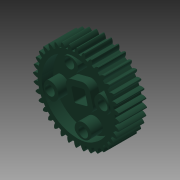
# Autodesk Inventor part: High Strength 36 Tooth Gear
Saved by Autodesk Inventor 2016 SP2 (Build 200236200, 236)
## iProperties
Category: Motion
Company: Autodesk Inc.
Created: 2012-02-19
Part Number: High Strength 36 Tooth Gear
Document SubType Name: Modeling
Designer: Autodesk Inc.
Density: 1.42 g/cm^3
Catalog Web Link: http://www.vexrobotics.com/276-2250.html
Description: 36 tooth spur gear
Vendor: VEX
Material: Acetal Resin, White
Mass: 10.4214 g
Surface Area: 82.0542 cm^2
Volume: 7.33901 cm^3
Appearance: VEX Gears Green
Author: Autodesk Inc.
Autodesk Inventor part; units mm, degrees
sketch "Sketch1" plane through (0, 0, 0) normal (0, 0, 1) x (1, 0, 0)
  arc A0 (-19.7463, 3.7758) -> (-19.8092, 3.4306) centre (0, 0) ccw
  arc A1 (-19.8092, 3.4306) -> (-17.8392, 2.2932) centre (-17.463, 5.2196) ccw
  arc A2 (-17.8392, 2.2932) -> (-17.9557, 1.0433) centre (0, 0) ccw
  arc A3 (-17.9557, 1.0433) -> (-20.102, 0.2896) centre (-18.1269, -1.9022) ccw
  arc A4 (-20.102, 0.2896) -> (-20.104, -0.0613) centre (0, 0) ccw
  arc A5 (-20.104, -0.0613) -> (-17.9664, -0.8393) centre (-18.1041, 2.1079) ccw
  arc A6 (-17.9664, -0.8393) -> (-17.8641, -2.0906) centre (0, 0) ccw
  arc A7 (-17.8641, -2.0906) -> (-19.8469, -3.2055) centre (-17.5212, -5.021) ccw
  arc A8 (-19.8469, -3.2055) -> (-19.7879, -3.5514) centre (0, 0) ccw
  arc A9 (-19.7879, -3.5514) -> (-17.5477, -3.9464) centre (-18.1951, -1.0679) ccw
  arc A10 (-17.5477, -3.9464) -> (-17.2297, -5.1609) centre (0, 0) ccw
  arc A11 (-17.2297, -5.1609) -> (-18.9887, -6.6032) centre (-16.3831, -7.9872) ccw
  arc A12 (-18.9887, -6.6032) -> (-18.8706, -6.9336) centre (0, 0) ccw
  arc A13 (-18.8706, -6.9336) -> (-16.5958, -6.9336) centre (-17.7332, -4.2112) ccw
  arc A14 (-16.5958, -6.9336) -> (-16.0717, -8.0744) centre (0, 0) ccw
  arc A15 (-16.0717, -8.0744) -> (-17.5536, -9.8002) centre (-14.7472, -10.7108) ccw
  arc A16 (-17.5536, -9.8002) -> (-17.3799, -10.1051) centre (0, 0) ccw
  arc A17 (-17.3799, -10.1051) -> (-15.1397, -9.7101) centre (-16.7325, -7.2266) ccw
  arc A18 (-15.1397, -9.7101) -> (-14.4255, -10.7425) centre (0, 0) ccw
  arc A19 (-14.4255, -10.7425) -> (-15.5852, -12.6995) centre (-12.6633, -13.1089) ccw
  arc A20 (-15.5852, -12.6995) -> (-15.3612, -12.9696) centre (0, 0) ccw
  arc A21 (-15.3612, -12.9696) -> (-13.2236, -12.1916) centre (-15.2235, -10.0223) ccw
  arc A22 (-13.2236, -12.1916) -> (-12.3409, -13.0843) centre (0, 0) ccw
  arc A23 (-12.3409, -13.0843) -> (-13.1431, -15.2129) centre (-10.1945, -15.1087) ccw
  arc A24 (-13.1431, -15.2129) -> (-12.8756, -15.44) centre (0, 0) ccw
  arc A25 (-12.8756, -15.44) -> (-10.9056, -14.3026) centre (-13.2518, -12.5136) ccw
  arc A26 (-10.9056, -14.3026) -> (-9.8814, -15.0285) centre (0, 0) ccw
  arc A27 (-9.8814, -15.0285) -> (-10.3018, -17.2641) centre (-7.4161, -16.6494) ccw
  arc A28 (-10.3018, -17.2641) -> (-9.9989, -17.4412) centre (0, 0) ccw
  arc A29 (-9.9989, -17.4412) -> (-8.2563, -15.979) centre (-10.8775, -14.6247) ccw
  arc A30 (-8.2563, -15.979) -> (-7.1216, -16.516) centre (0, 0) ccw
  arc A31 (-7.1216, -16.516) -> (-7.1474, -18.7907) centre (-4.4123, -17.6843) ccw
  arc A32 (-7.1474, -18.7907) -> (-6.8184, -18.9126) centre (0, 0) ccw
  arc A33 (-6.8184, -18.9126) -> (-5.3562, -17.17) centre (-8.1727, -16.2913) ccw
  arc A34 (-5.3562, -17.17) -> (-4.1454, -17.5018) centre (0, 0) ccw
  arc A35 (-4.1454, -17.5018) -> (-3.7758, -19.7463) centre (-1.2744, -18.1818) ccw
  arc A36 (-3.7758, -19.7463) -> (-3.4306, -19.8092) centre (0, 0) ccw
  arc A37 (-3.4306, -19.8092) -> (-2.2932, -17.8392) centre (-5.2196, -17.463) ccw
  arc A38 (-2.2932, -17.8392) -> (-1.0433, -17.9557) centre (0, 0) ccw
  arc A39 (-1.0433, -17.9557) -> (-0.2896, -20.102) centre (1.9022, -18.1269) ccw
  arc A40 (-0.2896, -20.102) -> (0.0613, -20.104) centre (0, 0) ccw
  arc A41 (0.0613, -20.104) -> (0.8393, -17.9664) centre (-2.1079, -18.1041) ccw
  arc A42 (0.8393, -17.9664) -> (2.0906, -17.8641) centre (0, 0) ccw
  arc A43 (2.0906, -17.8641) -> (3.2055, -19.8469) centre (5.021, -17.5212) ccw
  arc A44 (3.2055, -19.8469) -> (3.5514, -19.7879) centre (0, 0) ccw
  arc A45 (3.5514, -19.7879) -> (3.9464, -17.5477) centre (1.0679, -18.1951) ccw
  arc A46 (3.9464, -17.5477) -> (5.1609, -17.2297) centre (0, 0) ccw
  arc A47 (5.1609, -17.2297) -> (6.6032, -18.9887) centre (7.9872, -16.3831) ccw
  arc A48 (6.6032, -18.9887) -> (6.9336, -18.8706) centre (0, 0) ccw
  arc A49 (6.9336, -18.8706) -> (6.9336, -16.5958) centre (4.2112, -17.7332) ccw
  arc A50 (6.9336, -16.5958) -> (8.0744, -16.0717) centre (0, 0) ccw
  arc A51 (8.0744, -16.0717) -> (9.8002, -17.5536) centre (10.7108, -14.7472) ccw
  arc A52 (9.8002, -17.5536) -> (10.1051, -17.3799) centre (0, 0) ccw
  arc A53 (10.1051, -17.3799) -> (9.7101, -15.1397) centre (7.2266, -16.7325) ccw
  arc A54 (9.7101, -15.1397) -> (10.7425, -14.4255) centre (0, 0) ccw
  arc A55 (10.7425, -14.4255) -> (12.6995, -15.5852) centre (13.1089, -12.6633) ccw
  arc A56 (12.6995, -15.5852) -> (12.9696, -15.3612) centre (0, 0) ccw
  arc A57 (12.9696, -15.3612) -> (12.1916, -13.2236) centre (10.0223, -15.2235) ccw
  arc A58 (12.1916, -13.2236) -> (13.0843, -12.3409) centre (0, 0) ccw
  arc A59 (13.0843, -12.3409) -> (15.2129, -13.1431) centre (15.1087, -10.1945) ccw
  arc A60 (15.2129, -13.1431) -> (15.44, -12.8756) centre (0, 0) ccw
  arc A61 (15.44, -12.8756) -> (14.3026, -10.9056) centre (12.5136, -13.2518) ccw
  arc A62 (14.3026, -10.9056) -> (15.0285, -9.8814) centre (0, 0) ccw
  arc A63 (15.0285, -9.8814) -> (17.2641, -10.3018) centre (16.6494, -7.4161) ccw
  arc A64 (17.2641, -10.3018) -> (17.4412, -9.9989) centre (0, 0) ccw
  arc A65 (17.4412, -9.9989) -> (15.979, -8.2563) centre (14.6247, -10.8775) ccw
  arc A66 (15.979, -8.2563) -> (16.516, -7.1216) centre (0, 0) ccw
  arc A67 (16.516, -7.1216) -> (18.7907, -7.1474) centre (17.6843, -4.4123) ccw
  arc A68 (18.7907, -7.1474) -> (18.9126, -6.8184) centre (0, 0) ccw
  arc A69 (18.9126, -6.8184) -> (17.17, -5.3562) centre (16.2913, -8.1727) ccw
  arc A70 (17.17, -5.3562) -> (17.5018, -4.1454) centre (0, 0) ccw
  arc A71 (17.5018, -4.1454) -> (19.7463, -3.7758) centre (18.1818, -1.2744) ccw
  arc A72 (19.7463, -3.7758) -> (19.8092, -3.4306) centre (0, 0) ccw
  arc A73 (19.8092, -3.4306) -> (17.8392, -2.2932) centre (17.463, -5.2196) ccw
  arc A74 (17.8392, -2.2932) -> (17.9557, -1.0433) centre (0, 0) ccw
  arc A75 (17.9557, -1.0433) -> (20.102, -0.2896) centre (18.1269, 1.9022) ccw
  arc A76 (20.102, -0.2896) -> (20.104, 0.0613) centre (0, 0) ccw
  arc A77 (20.104, 0.0613) -> (17.9664, 0.8393) centre (18.1041, -2.1079) ccw
  arc A78 (17.9664, 0.8393) -> (17.8641, 2.0906) centre (0, 0) ccw
  arc A79 (17.8641, 2.0906) -> (19.8469, 3.2055) centre (17.5212, 5.021) ccw
  arc A80 (19.8469, 3.2055) -> (19.7879, 3.5514) centre (0, 0) ccw
  arc A81 (19.7879, 3.5514) -> (17.5477, 3.9464) centre (18.1951, 1.0679) ccw
  arc A82 (17.5477, 3.9464) -> (17.2297, 5.1609) centre (0, 0) ccw
  arc A83 (17.2297, 5.1609) -> (18.9887, 6.6032) centre (16.3831, 7.9872) ccw
  arc A84 (18.9887, 6.6032) -> (18.8706, 6.9336) centre (0, 0) ccw
  arc A85 (18.8706, 6.9336) -> (16.5958, 6.9336) centre (17.7332, 4.2112) ccw
  arc A86 (16.5958, 6.9336) -> (16.0717, 8.0744) centre (0, 0) ccw
  arc A87 (16.0717, 8.0744) -> (17.5536, 9.8002) centre (14.7472, 10.7108) ccw
  arc A88 (17.5536, 9.8002) -> (17.3799, 10.1051) centre (0, 0) ccw
  arc A89 (17.3799, 10.1051) -> (15.1397, 9.7101) centre (16.7325, 7.2266) ccw
  arc A90 (15.1397, 9.7101) -> (14.4255, 10.7425) centre (0, 0) ccw
  arc A91 (14.4255, 10.7425) -> (15.5852, 12.6995) centre (12.6633, 13.1089) ccw
  arc A92 (15.5852, 12.6995) -> (15.3612, 12.9696) centre (0, 0) ccw
  arc A93 (15.3612, 12.9696) -> (13.2235, 12.1916) centre (15.2235, 10.0223) ccw
  arc A94 (13.2235, 12.1916) -> (12.3409, 13.0843) centre (0, 0) ccw
  arc A95 (12.3409, 13.0843) -> (13.1431, 15.2129) centre (10.1945, 15.1087) ccw
  arc A96 (13.1431, 15.2129) -> (12.8756, 15.44) centre (0, 0) ccw
  arc A97 (12.8756, 15.44) -> (10.9056, 14.3026) centre (13.2518, 12.5136) ccw
  arc A98 (10.9056, 14.3026) -> (9.8814, 15.0285) centre (0, 0) ccw
  arc A99 (9.8814, 15.0285) -> (10.3018, 17.2641) centre (7.4161, 16.6494) ccw
  arc A100 (10.3018, 17.2641) -> (9.9989, 17.4412) centre (0, 0) ccw
  arc A101 (9.9989, 17.4412) -> (8.2563, 15.979) centre (10.8775, 14.6247) ccw
  arc A102 (8.2563, 15.979) -> (7.1216, 16.516) centre (0, 0) ccw
  arc A103 (7.1216, 16.516) -> (7.1474, 18.7907) centre (4.4123, 17.6843) ccw
  arc A104 (7.1474, 18.7907) -> (6.8184, 18.9126) centre (0, 0) ccw
  arc A105 (6.8184, 18.9126) -> (5.3562, 17.17) centre (8.1727, 16.2913) ccw
  arc A106 (5.3562, 17.17) -> (4.1454, 17.5018) centre (0, 0) ccw
  arc A107 (4.1454, 17.5018) -> (3.7758, 19.7463) centre (1.2744, 18.1818) ccw
  arc A108 (3.7758, 19.7463) -> (3.4306, 19.8092) centre (0, 0) ccw
  arc A109 (3.4306, 19.8092) -> (2.2932, 17.8392) centre (5.2196, 17.463) ccw
  arc A110 (2.2932, 17.8392) -> (1.0433, 17.9557) centre (0, 0) ccw
  arc A111 (1.0433, 17.9557) -> (0.2896, 20.102) centre (-1.9022, 18.1269) ccw
  arc A112 (0.2896, 20.102) -> (-0.0613, 20.104) centre (0, 0) ccw
  arc A113 (-0.0613, 20.104) -> (-0.8393, 17.9664) centre (2.1079, 18.1041) ccw
  arc A114 (-0.8393, 17.9664) -> (-2.0906, 17.8641) centre (0, 0) ccw
  arc A115 (-2.0906, 17.8641) -> (-3.2055, 19.8469) centre (-5.021, 17.5212) ccw
  arc A116 (-3.2055, 19.8469) -> (-3.5514, 19.7879) centre (0, 0) ccw
  arc A117 (-3.5514, 19.7879) -> (-3.9464, 17.5477) centre (-1.0679, 18.1951) ccw
  arc A118 (-3.9464, 17.5477) -> (-5.1609, 17.2297) centre (0, 0) ccw
  arc A119 (-5.1609, 17.2297) -> (-6.6032, 18.9888) centre (-7.9872, 16.3831) ccw
  arc A120 (-6.6032, 18.9888) -> (-6.9336, 18.8706) centre (0, 0) ccw
  arc A121 (-6.9336, 18.8706) -> (-6.9336, 16.5958) centre (-4.2112, 17.7332) ccw
  arc A122 (-6.9336, 16.5958) -> (-8.0744, 16.0717) centre (0, 0) ccw
  arc A123 (-8.0744, 16.0717) -> (-9.8002, 17.5536) centre (-10.7108, 14.7472) ccw
  arc A124 (-9.8002, 17.5536) -> (-10.1051, 17.3799) centre (0, 0) ccw
  arc A125 (-10.1051, 17.3799) -> (-9.7101, 15.1397) centre (-7.2266, 16.7325) ccw
  arc A126 (-9.7101, 15.1397) -> (-10.7425, 14.4255) centre (0, 0) ccw
  arc A127 (-10.7425, 14.4255) -> (-12.6995, 15.5852) centre (-13.1089, 12.6633) ccw
  arc A128 (-12.6995, 15.5852) -> (-12.9696, 15.3612) centre (0, 0) ccw
  arc A129 (-12.9696, 15.3612) -> (-12.1916, 13.2236) centre (-10.0223, 15.2235) ccw
  arc A130 (-12.1916, 13.2236) -> (-13.0843, 12.3409) centre (0, 0) ccw
  arc A131 (-13.0843, 12.3409) -> (-15.2129, 13.1431) centre (-15.1087, 10.1945) ccw
  arc A132 (-15.2129, 13.1431) -> (-15.44, 12.8756) centre (0, 0) ccw
  arc A133 (-15.44, 12.8756) -> (-14.3026, 10.9056) centre (-12.5136, 13.2518) ccw
  arc A134 (-14.3026, 10.9056) -> (-15.0285, 9.8814) centre (0, 0) ccw
  arc A135 (-15.0285, 9.8814) -> (-17.2641, 10.3018) centre (-16.6494, 7.4161) ccw
  arc A136 (-17.2641, 10.3018) -> (-17.4412, 9.9989) centre (0, 0) ccw
  arc A137 (-17.4412, 9.9989) -> (-15.979, 8.2563) centre (-14.6247, 10.8775) ccw
  arc A138 (-15.979, 8.2563) -> (-16.516, 7.1216) centre (0, 0) ccw
  arc A139 (-16.516, 7.1216) -> (-18.7907, 7.1474) centre (-17.6843, 4.4123) ccw
  arc A140 (-18.7907, 7.1474) -> (-18.9126, 6.8184) centre (0, 0) ccw
  arc A141 (-18.9126, 6.8184) -> (-17.17, 5.3562) centre (-16.2913, 8.1727) ccw
  arc A142 (-17.17, 5.3562) -> (-17.5018, 4.1454) centre (0, 0) ccw
  arc A143 (-17.5018, 4.1454) -> (-19.7463, 3.7758) centre (-18.1818, 1.2744) ccw
  arc A144 (-8.6835, 13.422) -> (-15.9553, 0.9903) centre (0, 0) ccw
  arc A145 (0.9903, 15.9553) -> (-8.6835, 13.422) centre (-0.8133, 3.1059) ccw
  arc A146 (13.422, 8.6835) -> (0.9903, 15.9553) centre (0, 0) ccw
  arc A147 (15.9553, -0.9903) -> (13.422, 8.6835) centre (3.1059, 0.8133) ccw
  arc A148 (8.6835, -13.422) -> (15.9553, -0.9903) centre (0, 0) ccw
  arc A149 (-0.9903, -15.9553) -> (8.6835, -13.422) centre (0.8133, -3.1059) ccw
  arc A150 (-13.422, -8.6835) -> (-0.9903, -15.9553) centre (0, 0) ccw
  arc A151 (-15.9553, 0.9903) -> (-13.422, -8.6835) centre (-3.1059, -0.8133) ccw
  line L0 (0.9929, 6.2349) -> (-3.9214, 4.948)
  arc A152 (-3.9214, 4.948) -> (-6.2349, 0.9929) centre (-3.1006, 1.8137) ccw
  line L1 (-6.2349, 0.9929) -> (-4.948, -3.9214)
  arc A153 (-4.948, -3.9214) -> (-0.9929, -6.2349) centre (-1.8137, -3.1006) ccw
  line L2 (-0.9929, -6.2349) -> (3.9214, -4.948)
  arc A154 (3.9214, -4.948) -> (6.2349, -0.9929) centre (3.1006, -1.8137) ccw
  line L3 (6.2349, -0.9929) -> (4.948, 3.9214)
  arc A155 (4.948, 3.9214) -> (0.9929, 6.2349) centre (1.8137, 3.1006) ccw
  arc A156 (-3.2615, 2.428) -> (-3.7149, 1.6528) centre (-3.1006, 1.8137) ccw
  line L4 (-3.2615, 2.428) -> (1.6528, 3.7149)
  arc A157 (2.428, 3.2615) -> (1.6528, 3.7149) centre (1.8137, 3.1006) ccw
  line L5 (2.428, 3.2615) -> (3.7149, -1.6528)
  arc A158 (3.2615, -2.428) -> (3.7149, -1.6528) centre (3.1006, -1.8137) ccw
  line L6 (3.2615, -2.428) -> (-1.6528, -3.7149)
  arc A159 (-2.428, -3.2615) -> (-1.6528, -3.7149) centre (-1.8137, -3.1006) ccw
  line L7 (-2.428, -3.2615) -> (-3.7149, 1.6528)
  arc A160 (-0.6522, -13.299) -> (7.0868, -11.2724) centre (2.8806, -11.0001) ccw
  arc A161 (7.0868, -11.2724) -> (-0.6522, -13.299) centre (3.2173, -12.2857) ccw
  circle A162 centre (3.2173, -12.2857) radius 2.2225
  arc A163 (-13.299, 0.6522) -> (-11.2724, -7.0868) centre (-11.0001, -2.8806) ccw
  arc A164 (-11.2724, -7.0868) -> (-13.299, 0.6522) centre (-12.2857, -3.2173) ccw
  circle A165 centre (-12.2857, -3.2173) radius 2.2225
  arc A166 (0.6522, 13.299) -> (-7.0868, 11.2724) centre (-2.8806, 11.0001) ccw
  arc A167 (-7.0868, 11.2724) -> (0.6522, 13.299) centre (-3.2173, 12.2857) ccw
  circle A168 centre (-3.2173, 12.2857) radius 2.2225
  arc A169 (13.299, -0.6522) -> (11.2724, 7.0868) centre (11.0001, 2.8806) ccw
  arc A170 (11.2724, 7.0868) -> (13.299, -0.6522) centre (12.2857, 3.2173) ccw
  circle A171 centre (12.2857, 3.2173) radius 2.2225
  point P0 (0, 0)
  constraints: 336 point on circle, 172 centre point, 16 end point
extrude "Extrusion1" add sketch "Sketch1" against normal blind 12.7 contours A143 A142 A141 A140 A139 A138 A137 A136 A135 A134 A133 A132 A131 A130 A129 A128 A127 A126 A125 A124 A123 A122 A121 A120 A119 A118 A117 A116 A115 A114 A113 A112 A111 A110 A109 A108 A107 A106 A105 A104 A103 A102 A101 A100 A99 A98 A97 A96 A95 A94 A93 A92 A91 A90 A89 A88 A87 A86 A85 A84 A83 A82 A81 A80 A79 A78 A77 A76 A75 A74 A73 A72 A71 A70 A69 A68 A67 A66 A65 A64 A63 A62 A61 A60 A59 A58 A57 A56 A55 A54 A53 A52 A51 A50 A49 A48 A47 A46 A45 A44 A43 A42 A41 A40 A39 A38 A37 A36 A35 A34 A33 A32 A31 A30 A29 A28 A27 A26 A25 A24 A23 A22 A21 A20 A19 A18 A17 A16 A15 A14 A13 A12 A11 A10 A9 A8 A7 A6 A5 A4 A3 A2 A1 A0
ref_plane "Work Plane1" through (0, 0, -6.35) normal (0, 0, 1) x (1, 0, 0)
sketch "Sketch2" plane through (0, 0, -6.35) normal (0, 0, 1) x (1, 0, 0)
  arc A0 (-15.9553, 0.9903) -> (-13.422, -8.6835) centre (-3.1059, -0.8133) ccw projected
  arc A1 (-13.422, -8.6835) -> (-0.9903, -15.9553) centre (0, 0) ccw projected
  arc A2 (-0.9903, -15.9553) -> (8.6835, -13.422) centre (0.8133, -3.1059) ccw projected
  arc A3 (8.6835, -13.422) -> (15.9553, -0.9903) centre (0, 0) ccw projected
  arc A4 (15.9553, -0.9903) -> (13.422, 8.6835) centre (3.1059, 0.8133) ccw projected
  arc A5 (13.422, 8.6835) -> (0.9903, 15.9553) centre (0, 0) ccw projected
  arc A6 (0.9903, 15.9553) -> (-8.6835, 13.422) centre (-0.8133, 3.1059) ccw projected
  arc A7 (-8.6835, 13.422) -> (-15.9553, 0.9903) centre (0, 0) ccw projected
  arc A8 (-15.979, 8.2563) -> (-16.516, 7.1216) centre (0, 0) ccw projected
  arc A9 (-17.4412, 9.9989) -> (-15.979, 8.2563) centre (-14.6247, 10.8775) ccw projected
  arc A10 (-17.2641, 10.3018) -> (-17.4412, 9.9989) centre (0, 0) ccw projected
  arc A11 (-15.0285, 9.8814) -> (-17.2641, 10.3018) centre (-16.6494, 7.4161) ccw projected
  arc A12 (-14.3026, 10.9056) -> (-15.0285, 9.8814) centre (0, 0) ccw projected
  arc A13 (-15.44, 12.8756) -> (-14.3026, 10.9056) centre (-12.5136, 13.2518) ccw projected
  arc A14 (-15.2129, 13.1431) -> (-15.44, 12.8756) centre (0, 0) ccw projected
  arc A15 (-13.0843, 12.3409) -> (-15.2129, 13.1431) centre (-15.1087, 10.1945) ccw projected
  arc A16 (-12.1916, 13.2236) -> (-13.0843, 12.3409) centre (0, 0) ccw projected
  arc A17 (-12.9696, 15.3612) -> (-12.1916, 13.2236) centre (-10.0223, 15.2235) ccw projected
  arc A18 (-12.6995, 15.5852) -> (-12.9696, 15.3612) centre (0, 0) ccw projected
  arc A19 (-10.7425, 14.4255) -> (-12.6995, 15.5852) centre (-13.1089, 12.6633) ccw projected
  arc A20 (-9.7101, 15.1397) -> (-10.7425, 14.4255) centre (0, 0) ccw projected
  arc A21 (-10.1051, 17.3799) -> (-9.7101, 15.1397) centre (-7.2266, 16.7325) ccw projected
  arc A22 (-9.8002, 17.5536) -> (-10.1051, 17.3799) centre (0, 0) ccw projected
  arc A23 (-8.0744, 16.0717) -> (-9.8002, 17.5536) centre (-10.7108, 14.7472) ccw projected
  arc A24 (-6.9336, 16.5958) -> (-8.0744, 16.0717) centre (0, 0) ccw projected
  arc A25 (-6.9336, 18.8706) -> (-6.9336, 16.5958) centre (-4.2112, 17.7332) ccw projected
  arc A26 (-6.6032, 18.9888) -> (-6.9336, 18.8706) centre (0, 0) ccw projected
  arc A27 (-5.1609, 17.2297) -> (-6.6032, 18.9888) centre (-7.9872, 16.3831) ccw projected
  arc A28 (-3.9464, 17.5477) -> (-5.1609, 17.2297) centre (0, 0) ccw projected
  arc A29 (-3.5514, 19.7879) -> (-3.9464, 17.5477) centre (-1.0679, 18.1951) ccw projected
  arc A30 (-3.2055, 19.8469) -> (-3.5514, 19.7879) centre (0, 0) ccw projected
  arc A31 (-2.0906, 17.8641) -> (-3.2055, 19.8469) centre (-5.021, 17.5212) ccw projected
  arc A32 (-0.8393, 17.9664) -> (-2.0906, 17.8641) centre (0, 0) ccw projected
  arc A33 (-0.0613, 20.104) -> (-0.8393, 17.9664) centre (2.1079, 18.1041) ccw projected
  arc A34 (0.2896, 20.102) -> (-0.0613, 20.104) centre (0, 0) ccw projected
  arc A35 (1.0433, 17.9557) -> (0.2896, 20.102) centre (-1.9022, 18.1269) ccw projected
  arc A36 (2.2932, 17.8392) -> (1.0433, 17.9557) centre (0, 0) ccw projected
  arc A37 (3.4306, 19.8092) -> (2.2932, 17.8392) centre (5.2196, 17.463) ccw projected
  arc A38 (3.7758, 19.7463) -> (3.4306, 19.8092) centre (0, 0) ccw projected
  arc A39 (4.1454, 17.5018) -> (3.7758, 19.7463) centre (1.2744, 18.1818) ccw projected
  arc A40 (5.3562, 17.17) -> (4.1454, 17.5018) centre (0, 0) ccw projected
  arc A41 (6.8184, 18.9126) -> (5.3562, 17.17) centre (8.1727, 16.2913) ccw projected
  arc A42 (7.1474, 18.7907) -> (6.8184, 18.9126) centre (0, 0) ccw projected
  arc A43 (7.1216, 16.516) -> (7.1474, 18.7907) centre (4.4123, 17.6843) ccw projected
  arc A44 (8.2563, 15.979) -> (7.1216, 16.516) centre (0, 0) ccw projected
  arc A45 (9.9989, 17.4412) -> (8.2563, 15.979) centre (10.8775, 14.6247) ccw projected
  arc A46 (10.3018, 17.2641) -> (9.9989, 17.4412) centre (0, 0) ccw projected
  arc A47 (9.8814, 15.0285) -> (10.3018, 17.2641) centre (7.4161, 16.6494) ccw projected
  arc A48 (10.9056, 14.3026) -> (9.8814, 15.0285) centre (0, 0) ccw projected
  arc A49 (12.8756, 15.44) -> (10.9056, 14.3026) centre (13.2518, 12.5136) ccw projected
  arc A50 (13.1431, 15.2129) -> (12.8756, 15.44) centre (0, 0) ccw projected
  arc A51 (12.3409, 13.0843) -> (13.1431, 15.2129) centre (10.1945, 15.1087) ccw projected
  arc A52 (13.2235, 12.1916) -> (12.3409, 13.0843) centre (0, 0) ccw projected
  arc A53 (15.3612, 12.9696) -> (13.2235, 12.1916) centre (15.2235, 10.0223) ccw projected
  arc A54 (15.5852, 12.6995) -> (15.3612, 12.9696) centre (0, 0) ccw projected
  arc A55 (14.4255, 10.7425) -> (15.5852, 12.6995) centre (12.6633, 13.1089) ccw projected
  arc A56 (15.1397, 9.7101) -> (14.4255, 10.7425) centre (0, 0) ccw projected
  arc A57 (17.3799, 10.1051) -> (15.1397, 9.7101) centre (16.7325, 7.2266) ccw projected
  arc A58 (17.5536, 9.8002) -> (17.3799, 10.1051) centre (0, 0) ccw projected
  arc A59 (16.0717, 8.0744) -> (17.5536, 9.8002) centre (14.7472, 10.7108) ccw projected
  arc A60 (16.5958, 6.9336) -> (16.0717, 8.0744) centre (0, 0) ccw projected
  arc A61 (18.8706, 6.9336) -> (16.5958, 6.9336) centre (17.7332, 4.2112) ccw projected
  arc A62 (18.9887, 6.6032) -> (18.8706, 6.9336) centre (0, 0) ccw projected
  arc A63 (17.2297, 5.1609) -> (18.9887, 6.6032) centre (16.3831, 7.9872) ccw projected
  arc A64 (17.5477, 3.9464) -> (17.2297, 5.1609) centre (0, 0) ccw projected
  arc A65 (19.7879, 3.5514) -> (17.5477, 3.9464) centre (18.1951, 1.0679) ccw projected
  arc A66 (19.8469, 3.2055) -> (19.7879, 3.5514) centre (0, 0) ccw projected
  arc A67 (17.8641, 2.0906) -> (19.8469, 3.2055) centre (17.5212, 5.021) ccw projected
  arc A68 (17.9664, 0.8393) -> (17.8641, 2.0906) centre (0, 0) ccw projected
  arc A69 (20.104, 0.0613) -> (17.9664, 0.8393) centre (18.1041, -2.1079) ccw projected
  arc A70 (20.102, -0.2896) -> (20.104, 0.0613) centre (0, 0) ccw projected
  arc A71 (17.9557, -1.0433) -> (20.102, -0.2896) centre (18.1269, 1.9022) ccw projected
  arc A72 (17.8392, -2.2932) -> (17.9557, -1.0433) centre (0, 0) ccw projected
  arc A73 (19.8092, -3.4306) -> (17.8392, -2.2932) centre (17.463, -5.2196) ccw projected
  arc A74 (19.7463, -3.7758) -> (19.8092, -3.4306) centre (0, 0) ccw projected
  arc A75 (17.5018, -4.1454) -> (19.7463, -3.7758) centre (18.1818, -1.2744) ccw projected
  arc A76 (17.17, -5.3562) -> (17.5018, -4.1454) centre (0, 0) ccw projected
  arc A77 (18.9126, -6.8184) -> (17.17, -5.3562) centre (16.2913, -8.1727) ccw projected
  arc A78 (18.7907, -7.1474) -> (18.9126, -6.8184) centre (0, 0) ccw projected
  arc A79 (16.516, -7.1216) -> (18.7907, -7.1474) centre (17.6843, -4.4123) ccw projected
  arc A80 (15.979, -8.2563) -> (16.516, -7.1216) centre (0, 0) ccw projected
  arc A81 (17.4412, -9.9989) -> (15.979, -8.2563) centre (14.6247, -10.8775) ccw projected
  arc A82 (17.2641, -10.3018) -> (17.4412, -9.9989) centre (0, 0) ccw projected
  arc A83 (15.0285, -9.8814) -> (17.2641, -10.3018) centre (16.6494, -7.4161) ccw projected
  arc A84 (14.3026, -10.9056) -> (15.0285, -9.8814) centre (0, 0) ccw projected
  arc A85 (15.44, -12.8756) -> (14.3026, -10.9056) centre (12.5136, -13.2518) ccw projected
  arc A86 (15.2129, -13.1431) -> (15.44, -12.8756) centre (0, 0) ccw projected
  arc A87 (13.0843, -12.3409) -> (15.2129, -13.1431) centre (15.1087, -10.1945) ccw projected
  arc A88 (12.1916, -13.2236) -> (13.0843, -12.3409) centre (0, 0) ccw projected
  arc A89 (12.9696, -15.3612) -> (12.1916, -13.2236) centre (10.0223, -15.2235) ccw projected
  arc A90 (12.6995, -15.5852) -> (12.9696, -15.3612) centre (0, 0) ccw projected
  arc A91 (10.7425, -14.4255) -> (12.6995, -15.5852) centre (13.1089, -12.6633) ccw projected
  arc A92 (9.7101, -15.1397) -> (10.7425, -14.4255) centre (0, 0) ccw projected
  arc A93 (10.1051, -17.3799) -> (9.7101, -15.1397) centre (7.2266, -16.7325) ccw projected
  arc A94 (9.8002, -17.5536) -> (10.1051, -17.3799) centre (0, 0) ccw projected
  arc A95 (8.0744, -16.0717) -> (9.8002, -17.5536) centre (10.7108, -14.7472) ccw projected
  arc A96 (6.9336, -16.5958) -> (8.0744, -16.0717) centre (0, 0) ccw projected
  arc A97 (6.9336, -18.8706) -> (6.9336, -16.5958) centre (4.2112, -17.7332) ccw projected
  arc A98 (6.6032, -18.9887) -> (6.9336, -18.8706) centre (0, 0) ccw projected
  arc A99 (5.1609, -17.2297) -> (6.6032, -18.9887) centre (7.9872, -16.3831) ccw projected
  arc A100 (3.9464, -17.5477) -> (5.1609, -17.2297) centre (0, 0) ccw projected
  arc A101 (3.5514, -19.7879) -> (3.9464, -17.5477) centre (1.0679, -18.1951) ccw projected
  arc A102 (3.2055, -19.8469) -> (3.5514, -19.7879) centre (0, 0) ccw projected
  arc A103 (2.0906, -17.8641) -> (3.2055, -19.8469) centre (5.021, -17.5212) ccw projected
  arc A104 (0.8393, -17.9664) -> (2.0906, -17.8641) centre (0, 0) ccw projected
  arc A105 (0.0613, -20.104) -> (0.8393, -17.9664) centre (-2.1079, -18.1041) ccw projected
  arc A106 (-0.2896, -20.102) -> (0.0613, -20.104) centre (0, 0) ccw projected
  arc A107 (-1.0433, -17.9557) -> (-0.2896, -20.102) centre (1.9022, -18.1269) ccw projected
  arc A108 (-2.2932, -17.8392) -> (-1.0433, -17.9557) centre (0, 0) ccw projected
  arc A109 (-3.4306, -19.8092) -> (-2.2932, -17.8392) centre (-5.2196, -17.463) ccw projected
  arc A110 (-3.7758, -19.7463) -> (-3.4306, -19.8092) centre (0, 0) ccw projected
  arc A111 (-4.1454, -17.5018) -> (-3.7758, -19.7463) centre (-1.2744, -18.1818) ccw projected
  arc A112 (-5.3562, -17.17) -> (-4.1454, -17.5018) centre (0, 0) ccw projected
  arc A113 (-6.8184, -18.9126) -> (-5.3562, -17.17) centre (-8.1727, -16.2913) ccw projected
  arc A114 (-7.1474, -18.7907) -> (-6.8184, -18.9126) centre (0, 0) ccw projected
  arc A115 (-7.1216, -16.516) -> (-7.1474, -18.7907) centre (-4.4123, -17.6843) ccw projected
  arc A116 (-8.2563, -15.979) -> (-7.1216, -16.516) centre (0, 0) ccw projected
  arc A117 (-9.9989, -17.4412) -> (-8.2563, -15.979) centre (-10.8775, -14.6247) ccw projected
  arc A118 (-10.3018, -17.2641) -> (-9.9989, -17.4412) centre (0, 0) ccw projected
  arc A119 (-9.8814, -15.0285) -> (-10.3018, -17.2641) centre (-7.4161, -16.6494) ccw projected
  arc A120 (-10.9056, -14.3026) -> (-9.8814, -15.0285) centre (0, 0) ccw projected
  arc A121 (-12.8756, -15.44) -> (-10.9056, -14.3026) centre (-13.2518, -12.5136) ccw projected
  arc A122 (-13.1431, -15.2129) -> (-12.8756, -15.44) centre (0, 0) ccw projected
  arc A123 (-12.3409, -13.0843) -> (-13.1431, -15.2129) centre (-10.1945, -15.1087) ccw projected
  arc A124 (-13.2236, -12.1916) -> (-12.3409, -13.0843) centre (0, 0) ccw projected
  arc A125 (-15.3612, -12.9696) -> (-13.2236, -12.1916) centre (-15.2235, -10.0223) ccw projected
  arc A126 (-15.5852, -12.6995) -> (-15.3612, -12.9696) centre (0, 0) ccw projected
  arc A127 (-14.4255, -10.7425) -> (-15.5852, -12.6995) centre (-12.6633, -13.1089) ccw projected
  arc A128 (-15.1397, -9.7101) -> (-14.4255, -10.7425) centre (0, 0) ccw projected
  arc A129 (-17.3799, -10.1051) -> (-15.1397, -9.7101) centre (-16.7325, -7.2266) ccw projected
  arc A130 (-17.5536, -9.8002) -> (-17.3799, -10.1051) centre (0, 0) ccw projected
  arc A131 (-16.0717, -8.0744) -> (-17.5536, -9.8002) centre (-14.7472, -10.7108) ccw projected
  arc A132 (-16.5958, -6.9336) -> (-16.0717, -8.0744) centre (0, 0) ccw projected
  arc A133 (-18.8706, -6.9336) -> (-16.5958, -6.9336) centre (-17.7332, -4.2112) ccw projected
  arc A134 (-18.9887, -6.6032) -> (-18.8706, -6.9336) centre (0, 0) ccw projected
  arc A135 (-17.2297, -5.1609) -> (-18.9887, -6.6032) centre (-16.3831, -7.9872) ccw projected
  arc A136 (-17.5477, -3.9464) -> (-17.2297, -5.1609) centre (0, 0) ccw projected
  arc A137 (-19.7879, -3.5514) -> (-17.5477, -3.9464) centre (-18.1951, -1.0679) ccw projected
  arc A138 (-19.8469, -3.2055) -> (-19.7879, -3.5514) centre (0, 0) ccw projected
  arc A139 (-17.8641, -2.0906) -> (-19.8469, -3.2055) centre (-17.5212, -5.021) ccw projected
  arc A140 (-17.9664, -0.8393) -> (-17.8641, -2.0906) centre (0, 0) ccw projected
  arc A141 (-20.104, -0.0613) -> (-17.9664, -0.8393) centre (-18.1041, 2.1079) ccw projected
  arc A142 (-20.102, 0.2896) -> (-20.104, -0.0613) centre (0, 0) ccw projected
  arc A143 (-17.9557, 1.0433) -> (-20.102, 0.2896) centre (-18.1269, -1.9022) ccw projected
  arc A144 (-17.8392, 2.2932) -> (-17.9557, 1.0433) centre (0, 0) ccw projected
  arc A145 (-19.8092, 3.4306) -> (-17.8392, 2.2932) centre (-17.463, 5.2196) ccw projected
  arc A146 (-19.7463, 3.7758) -> (-19.8092, 3.4306) centre (0, 0) ccw projected
  arc A147 (-17.5018, 4.1454) -> (-19.7463, 3.7758) centre (-18.1818, 1.2744) ccw projected
  arc A148 (-17.17, 5.3562) -> (-17.5018, 4.1454) centre (0, 0) ccw projected
  arc A149 (-18.9126, 6.8184) -> (-17.17, 5.3562) centre (-16.2913, 8.1727) ccw projected
  arc A150 (-18.7907, 7.1474) -> (-18.9126, 6.8184) centre (0, 0) ccw projected
  arc A151 (-16.516, 7.1216) -> (-18.7907, 7.1474) centre (-17.6843, 4.4123) ccw projected
  point P0 (0, 0)
extrude "Extrusion2" add sketch "Sketch2" along normal mid plane 2.1844 contours A7 A6 A5 A4 A3 A2 A1 A0
extrude "Extrusion3" add sketch "Sketch1" against normal up to surface (12.7 mm away) contours A161 A160 | A164 A163 | A167 A166 | A170 A169
ref_plane "Work Plane2" through (0, 0, -1.47) normal (0, 0, 1) x (1, 0, 0)
ref_plane "Work Plane3" through (0, 0, -11.23) normal (0, 0, -1) x (-1, 0, 0)
extrude "Extrusion4" add sketch "Sketch1" against normal up to surface (9.76 mm away) from surface at -1.47 contours A155 L3 A154 L2 A153 L1 A152 L0
extrude "Extrusion5" cut sketch "Sketch1" against normal up to surface (12.7 mm away) contours A162 | A165 | A168 | A171
sketch "Sketch3" plane through (0, 0, 0) normal (0, 0, 1) x (1, 0, 0)
  arc A0 (-15.9553, 0.9903) -> (-13.422, -8.6835) centre (-3.1059, -0.8133) ccw projected
  arc A1 (-8.6835, 13.422) -> (-15.9553, 0.9903) centre (0, 0) ccw projected
  arc A2 (0.9903, 15.9553) -> (-8.6835, 13.422) centre (-0.8133, 3.1059) ccw projected
  arc A3 (13.422, 8.6835) -> (0.9903, 15.9553) centre (0, 0) ccw projected
  arc A4 (15.9553, -0.9903) -> (13.422, 8.6835) centre (3.1059, 0.8133) ccw projected
  arc A5 (8.6835, -13.422) -> (15.9553, -0.9903) centre (0, 0) ccw projected
  arc A6 (-0.9903, -15.9553) -> (8.6835, -13.422) centre (0.8133, -3.1059) ccw projected
  arc A7 (-13.422, -8.6835) -> (-0.9903, -15.9553) centre (0, 0) ccw projected
  arc A8 (-17.4412, 9.9989) -> (-15.979, 8.2563) centre (-14.6247, 10.8775) ccw projected
  arc A9 (-15.979, 8.2563) -> (-16.516, 7.1216) centre (0, 0) ccw projected
  arc A10 (-16.516, 7.1216) -> (-18.7907, 7.1474) centre (-17.6843, 4.4123) ccw projected
  arc A11 (-18.7907, 7.1474) -> (-18.9126, 6.8184) centre (0, 0) ccw projected
  arc A12 (-18.9126, 6.8184) -> (-17.17, 5.3562) centre (-16.2913, 8.1727) ccw projected
  arc A13 (-17.17, 5.3562) -> (-17.5018, 4.1454) centre (0, 0) ccw projected
  arc A14 (-17.5018, 4.1454) -> (-19.7463, 3.7758) centre (-18.1818, 1.2744) ccw projected
  arc A15 (-19.7463, 3.7758) -> (-19.8092, 3.4306) centre (0, 0) ccw projected
  arc A16 (-19.8092, 3.4306) -> (-17.8392, 2.2932) centre (-17.463, 5.2196) ccw projected
  arc A17 (-17.8392, 2.2932) -> (-17.9557, 1.0433) centre (0, 0) ccw projected
  arc A18 (-17.9557, 1.0433) -> (-20.102, 0.2896) centre (-18.1269, -1.9022) ccw projected
  arc A19 (-20.102, 0.2896) -> (-20.104, -0.0613) centre (0, 0) ccw projected
  arc A20 (-20.104, -0.0613) -> (-17.9664, -0.8393) centre (-18.1041, 2.1079) ccw projected
  arc A21 (-17.9664, -0.8393) -> (-17.8641, -2.0906) centre (0, 0) ccw projected
  arc A22 (-17.8641, -2.0906) -> (-19.8469, -3.2055) centre (-17.5212, -5.021) ccw projected
  arc A23 (-19.8469, -3.2055) -> (-19.7879, -3.5514) centre (0, 0) ccw projected
  arc A24 (-19.7879, -3.5514) -> (-17.5477, -3.9464) centre (-18.1951, -1.0679) ccw projected
  arc A25 (-17.5477, -3.9464) -> (-17.2297, -5.1609) centre (0, 0) ccw projected
  arc A26 (-17.2297, -5.1609) -> (-18.9887, -6.6032) centre (-16.3831, -7.9872) ccw projected
  arc A27 (-18.9887, -6.6032) -> (-18.8706, -6.9336) centre (0, 0) ccw projected
  arc A28 (-18.8706, -6.9336) -> (-16.5958, -6.9336) centre (-17.7332, -4.2112) ccw projected
  arc A29 (-16.5958, -6.9336) -> (-16.0717, -8.0744) centre (0, 0) ccw projected
  arc A30 (-16.0717, -8.0744) -> (-17.5536, -9.8002) centre (-14.7472, -10.7108) ccw projected
  arc A31 (-17.5536, -9.8002) -> (-17.3799, -10.1051) centre (0, 0) ccw projected
  arc A32 (-17.3799, -10.1051) -> (-15.1397, -9.7101) centre (-16.7325, -7.2266) ccw projected
  arc A33 (-15.1397, -9.7101) -> (-14.4255, -10.7425) centre (0, 0) ccw projected
  arc A34 (-14.4255, -10.7425) -> (-15.5852, -12.6995) centre (-12.6633, -13.1089) ccw projected
  arc A35 (-15.5852, -12.6995) -> (-15.3612, -12.9696) centre (0, 0) ccw projected
  arc A36 (-15.3612, -12.9696) -> (-13.2236, -12.1916) centre (-15.2235, -10.0223) ccw projected
  arc A37 (-13.2236, -12.1916) -> (-12.3409, -13.0843) centre (0, 0) ccw projected
  arc A38 (-12.3409, -13.0843) -> (-13.1431, -15.2129) centre (-10.1945, -15.1087) ccw projected
  arc A39 (-13.1431, -15.2129) -> (-12.8756, -15.44) centre (0, 0) ccw projected
  arc A40 (-12.8756, -15.44) -> (-10.9056, -14.3026) centre (-13.2518, -12.5136) ccw projected
  arc A41 (-10.9056, -14.3026) -> (-9.8814, -15.0285) centre (0, 0) ccw projected
  arc A42 (-9.8814, -15.0285) -> (-10.3018, -17.2641) centre (-7.4161, -16.6494) ccw projected
  arc A43 (-10.3018, -17.2641) -> (-9.9989, -17.4412) centre (0, 0) ccw projected
  arc A44 (-9.9989, -17.4412) -> (-8.2563, -15.979) centre (-10.8775, -14.6247) ccw projected
  arc A45 (-8.2563, -15.979) -> (-7.1216, -16.516) centre (0, 0) ccw projected
  arc A46 (-7.1216, -16.516) -> (-7.1474, -18.7907) centre (-4.4123, -17.6843) ccw projected
  arc A47 (-7.1474, -18.7907) -> (-6.8184, -18.9126) centre (0, 0) ccw projected
  arc A48 (-6.8184, -18.9126) -> (-5.3562, -17.17) centre (-8.1727, -16.2913) ccw projected
  arc A49 (-5.3562, -17.17) -> (-4.1454, -17.5018) centre (0, 0) ccw projected
  arc A50 (-4.1454, -17.5018) -> (-3.7758, -19.7463) centre (-1.2744, -18.1818) ccw projected
  arc A51 (-3.7758, -19.7463) -> (-3.4306, -19.8092) centre (0, 0) ccw projected
  arc A52 (-3.4306, -19.8092) -> (-2.2932, -17.8392) centre (-5.2196, -17.463) ccw projected
  arc A53 (-2.2932, -17.8392) -> (-1.0433, -17.9557) centre (0, 0) ccw projected
  arc A54 (-1.0433, -17.9557) -> (-0.2896, -20.102) centre (1.9022, -18.1269) ccw projected
  arc A55 (-0.2896, -20.102) -> (0.0613, -20.104) centre (0, 0) ccw projected
  arc A56 (0.0613, -20.104) -> (0.8393, -17.9664) centre (-2.1079, -18.1041) ccw projected
  arc A57 (0.8393, -17.9664) -> (2.0906, -17.8641) centre (0, 0) ccw projected
  arc A58 (2.0906, -17.8641) -> (3.2055, -19.8469) centre (5.021, -17.5212) ccw projected
  arc A59 (3.2055, -19.8469) -> (3.5514, -19.7879) centre (0, 0) ccw projected
  arc A60 (3.5514, -19.7879) -> (3.9464, -17.5477) centre (1.0679, -18.1951) ccw projected
  arc A61 (3.9464, -17.5477) -> (5.1609, -17.2297) centre (0, 0) ccw projected
  arc A62 (5.1609, -17.2297) -> (6.6032, -18.9887) centre (7.9872, -16.3831) ccw projected
  arc A63 (6.6032, -18.9887) -> (6.9336, -18.8706) centre (0, 0) ccw projected
  arc A64 (6.9336, -18.8706) -> (6.9336, -16.5958) centre (4.2112, -17.7332) ccw projected
  arc A65 (6.9336, -16.5958) -> (8.0744, -16.0717) centre (0, 0) ccw projected
  arc A66 (8.0744, -16.0717) -> (9.8002, -17.5536) centre (10.7108, -14.7472) ccw projected
  arc A67 (9.8002, -17.5536) -> (10.1051, -17.3799) centre (0, 0) ccw projected
  arc A68 (10.1051, -17.3799) -> (9.7101, -15.1397) centre (7.2266, -16.7325) ccw projected
  arc A69 (9.7101, -15.1397) -> (10.7425, -14.4255) centre (0, 0) ccw projected
  arc A70 (10.7425, -14.4255) -> (12.6995, -15.5852) centre (13.1089, -12.6633) ccw projected
  arc A71 (12.6995, -15.5852) -> (12.9696, -15.3612) centre (0, 0) ccw projected
  arc A72 (12.9696, -15.3612) -> (12.1916, -13.2236) centre (10.0223, -15.2235) ccw projected
  arc A73 (12.1916, -13.2236) -> (13.0843, -12.3409) centre (0, 0) ccw projected
  arc A74 (13.0843, -12.3409) -> (15.2129, -13.1431) centre (15.1087, -10.1945) ccw projected
  arc A75 (15.2129, -13.1431) -> (15.44, -12.8756) centre (0, 0) ccw projected
  arc A76 (15.44, -12.8756) -> (14.3026, -10.9056) centre (12.5136, -13.2518) ccw projected
  arc A77 (14.3026, -10.9056) -> (15.0285, -9.8814) centre (0, 0) ccw projected
  arc A78 (15.0285, -9.8814) -> (17.2641, -10.3018) centre (16.6494, -7.4161) ccw projected
  arc A79 (17.2641, -10.3018) -> (17.4412, -9.9989) centre (0, 0) ccw projected
  arc A80 (17.4412, -9.9989) -> (15.979, -8.2563) centre (14.6247, -10.8775) ccw projected
  arc A81 (15.979, -8.2563) -> (16.516, -7.1216) centre (0, 0) ccw projected
  arc A82 (16.516, -7.1216) -> (18.7907, -7.1474) centre (17.6843, -4.4123) ccw projected
  arc A83 (18.7907, -7.1474) -> (18.9126, -6.8184) centre (0, 0) ccw projected
  arc A84 (18.9126, -6.8184) -> (17.17, -5.3562) centre (16.2913, -8.1727) ccw projected
  arc A85 (17.17, -5.3562) -> (17.5018, -4.1454) centre (0, 0) ccw projected
  arc A86 (17.5018, -4.1454) -> (19.7463, -3.7758) centre (18.1818, -1.2744) ccw projected
  arc A87 (19.7463, -3.7758) -> (19.8092, -3.4306) centre (0, 0) ccw projected
  arc A88 (19.8092, -3.4306) -> (17.8392, -2.2932) centre (17.463, -5.2196) ccw projected
  arc A89 (17.8392, -2.2932) -> (17.9557, -1.0433) centre (0, 0) ccw projected
  arc A90 (17.9557, -1.0433) -> (20.102, -0.2896) centre (18.1269, 1.9022) ccw projected
  arc A91 (20.102, -0.2896) -> (20.104, 0.0613) centre (0, 0) ccw projected
  arc A92 (20.104, 0.0613) -> (17.9664, 0.8393) centre (18.1041, -2.1079) ccw projected
  arc A93 (17.9664, 0.8393) -> (17.8641, 2.0906) centre (0, 0) ccw projected
  arc A94 (17.8641, 2.0906) -> (19.8469, 3.2055) centre (17.5212, 5.021) ccw projected
  arc A95 (19.8469, 3.2055) -> (19.7879, 3.5514) centre (0, 0) ccw projected
  arc A96 (19.7879, 3.5514) -> (17.5477, 3.9464) centre (18.1951, 1.0679) ccw projected
  arc A97 (17.5477, 3.9464) -> (17.2297, 5.1609) centre (0, 0) ccw projected
  arc A98 (17.2297, 5.1609) -> (18.9887, 6.6032) centre (16.3831, 7.9872) ccw projected
  arc A99 (18.9887, 6.6032) -> (18.8706, 6.9336) centre (0, 0) ccw projected
  arc A100 (18.8706, 6.9336) -> (16.5958, 6.9336) centre (17.7332, 4.2112) ccw projected
  arc A101 (16.5958, 6.9336) -> (16.0717, 8.0744) centre (0, 0) ccw projected
  arc A102 (16.0717, 8.0744) -> (17.5536, 9.8002) centre (14.7472, 10.7108) ccw projected
  arc A103 (17.5536, 9.8002) -> (17.3799, 10.1051) centre (0, 0) ccw projected
  arc A104 (17.3799, 10.1051) -> (15.1397, 9.7101) centre (16.7325, 7.2266) ccw projected
  arc A105 (15.1397, 9.7101) -> (14.4255, 10.7425) centre (0, 0) ccw projected
  arc A106 (14.4255, 10.7425) -> (15.5852, 12.6995) centre (12.6633, 13.1089) ccw projected
  arc A107 (15.5852, 12.6995) -> (15.3612, 12.9696) centre (0, 0) ccw projected
  arc A108 (15.3612, 12.9696) -> (13.2235, 12.1916) centre (15.2235, 10.0223) ccw projected
  arc A109 (13.2235, 12.1916) -> (12.3409, 13.0843) centre (0, 0) ccw projected
  arc A110 (12.3409, 13.0843) -> (13.1431, 15.2129) centre (10.1945, 15.1087) ccw projected
  arc A111 (13.1431, 15.2129) -> (12.8756, 15.44) centre (0, 0) ccw projected
  arc A112 (12.8756, 15.44) -> (10.9056, 14.3026) centre (13.2518, 12.5136) ccw projected
  arc A113 (10.9056, 14.3026) -> (9.8814, 15.0285) centre (0, 0) ccw projected
  arc A114 (9.8814, 15.0285) -> (10.3018, 17.2641) centre (7.4161, 16.6494) ccw projected
  arc A115 (10.3018, 17.2641) -> (9.9989, 17.4412) centre (0, 0) ccw projected
  arc A116 (9.9989, 17.4412) -> (8.2563, 15.979) centre (10.8775, 14.6247) ccw projected
  arc A117 (8.2563, 15.979) -> (7.1216, 16.516) centre (0, 0) ccw projected
  arc A118 (7.1216, 16.516) -> (7.1474, 18.7907) centre (4.4123, 17.6843) ccw projected
  arc A119 (7.1474, 18.7907) -> (6.8184, 18.9126) centre (0, 0) ccw projected
  arc A120 (6.8184, 18.9126) -> (5.3562, 17.17) centre (8.1727, 16.2913) ccw projected
  arc A121 (5.3562, 17.17) -> (4.1454, 17.5018) centre (0, 0) ccw projected
  arc A122 (4.1454, 17.5018) -> (3.7758, 19.7463) centre (1.2744, 18.1818) ccw projected
  arc A123 (3.7758, 19.7463) -> (3.4306, 19.8092) centre (0, 0) ccw projected
  arc A124 (3.4306, 19.8092) -> (2.2932, 17.8392) centre (5.2196, 17.463) ccw projected
  arc A125 (2.2932, 17.8392) -> (1.0433, 17.9557) centre (0, 0) ccw projected
  arc A126 (1.0433, 17.9557) -> (0.2896, 20.102) centre (-1.9022, 18.1269) ccw projected
  arc A127 (0.2896, 20.102) -> (-0.0613, 20.104) centre (0, 0) ccw projected
  arc A128 (-0.0613, 20.104) -> (-0.8393, 17.9664) centre (2.1079, 18.1041) ccw projected
  arc A129 (-0.8393, 17.9664) -> (-2.0906, 17.8641) centre (0, 0) ccw projected
  arc A130 (-2.0906, 17.8641) -> (-3.2055, 19.8469) centre (-5.021, 17.5212) ccw projected
  arc A131 (-3.2055, 19.8469) -> (-3.5514, 19.7879) centre (0, 0) ccw projected
  arc A132 (-3.5514, 19.7879) -> (-3.9464, 17.5477) centre (-1.0679, 18.1951) ccw projected
  arc A133 (-3.9464, 17.5477) -> (-5.1609, 17.2297) centre (0, 0) ccw projected
  arc A134 (-5.1609, 17.2297) -> (-6.6032, 18.9888) centre (-7.9872, 16.3831) ccw projected
  arc A135 (-6.6032, 18.9888) -> (-6.9336, 18.8706) centre (0, 0) ccw projected
  arc A136 (-6.9336, 18.8706) -> (-6.9336, 16.5958) centre (-4.2112, 17.7332) ccw projected
  arc A137 (-6.9336, 16.5958) -> (-8.0744, 16.0717) centre (0, 0) ccw projected
  arc A138 (-8.0744, 16.0717) -> (-9.8002, 17.5536) centre (-10.7108, 14.7472) ccw projected
  arc A139 (-9.8002, 17.5536) -> (-10.1051, 17.3799) centre (0, 0) ccw projected
  arc A140 (-10.1051, 17.3799) -> (-9.7101, 15.1397) centre (-7.2266, 16.7325) ccw projected
  arc A141 (-9.7101, 15.1397) -> (-10.7425, 14.4255) centre (0, 0) ccw projected
  arc A142 (-10.7425, 14.4255) -> (-12.6995, 15.5852) centre (-13.1089, 12.6633) ccw projected
  arc A143 (-12.6995, 15.5852) -> (-12.9696, 15.3612) centre (0, 0) ccw projected
  arc A144 (-12.9696, 15.3612) -> (-12.1916, 13.2236) centre (-10.0223, 15.2235) ccw projected
  arc A145 (-12.1916, 13.2236) -> (-13.0843, 12.3409) centre (0, 0) ccw projected
  arc A146 (-13.0843, 12.3409) -> (-15.2129, 13.1431) centre (-15.1087, 10.1945) ccw projected
  arc A147 (-15.2129, 13.1431) -> (-15.44, 12.8756) centre (0, 0) ccw projected
  arc A148 (-15.44, 12.8756) -> (-14.3026, 10.9056) centre (-12.5136, 13.2518) ccw projected
  arc A149 (-14.3026, 10.9056) -> (-15.0285, 9.8814) centre (0, 0) ccw projected
  arc A150 (-15.0285, 9.8814) -> (-17.2641, 10.3018) centre (-16.6494, 7.4161) ccw projected
  arc A151 (-17.2641, 10.3018) -> (-17.4412, 9.9989) centre (0, 0) ccw projected
sketch "Sketch4" plane through (0, 0, -5.2578) normal (0, 0, 1) x (1, 0, 0)
  line L0 (-3.7149, 1.6528) -> (-2.428, -3.2615) projected
  arc A0 (-2.428, -3.2615) -> (-1.6528, -3.7149) centre (-1.8137, -3.1006) ccw projected
  line L1 (-1.6528, -3.7149) -> (3.2615, -2.428) projected
  arc A1 (3.2615, -2.428) -> (3.7149, -1.6528) centre (3.1006, -1.8137) ccw projected
  line L2 (3.7149, -1.6528) -> (2.428, 3.2615) projected
  arc A2 (2.428, 3.2615) -> (1.6528, 3.7149) centre (1.8137, 3.1006) ccw projected
  line L3 (1.6528, 3.7149) -> (-3.2615, 2.428) projected
  arc A3 (-3.2615, 2.428) -> (-3.7149, 1.6528) centre (-3.1006, 1.8137) ccw projected
  point P0 (0, 0)
extrude "Extrusion6" cut sketch "Sketch4" against normal up to surface (5.9722 mm away)
sketch "Sketch5" plane through (3.1006, -1.8137, -1.47) normal (0, 0, 1) x (0.863173, -0.5049082, 0)
  line L0 (-4.0411, 4.0411) -> (-7.6332, 0.449) projected
  circle A0 centre (-3.5921, 0) radius 3.175
  constraints: 1 centre point, 1 coincident, 1 tangent
surface extrude "ExtrusionSrf1" sketch "Sketch5" against normal up to surface (9.76 mm away) shown no curves A0
body "Solid1"
body "Srf1"
